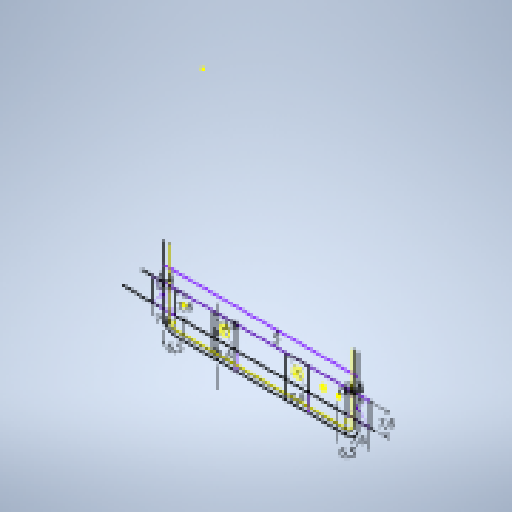
# Autodesk Inventor part: podstawa_rpi_board_2
Saved by Autodesk Inventor 2023.4 (Build 274418000, 418)
## iProperties
Created: 2024-09-15
Part Number: podstawa_rpi_board_2
Material: Generic
Document SubType Name: Modeling
Designer: komputer
Density: 1 g/cm^3
Appearance: Default
Author: komputer
Autodesk Inventor part; units mm, degrees
ref_plane "YZ Plane" through (0, 0, 0) normal (1, 0, 0) x (0, 1, 0)
ref_plane "XZ Plane" through (0, 0, 0) normal (0, 1, 0) x (-1, 0, 0)
ref_plane "XY Plane" through (0, 0, 0) normal (0, 0, 1) x (1, 0, 0)
sketch "Sketch1" plane through (0, 0, 0) normal (0, 0, 1) x (1, 0, 0)
  circle A0 centre (6.9875, -70.9975) radius 1.6 projected
  circle A1 centre (30.9875, -70.9975) radius 1.6 projected
  line L0 (49.2375, -55.2975) -> (49.2375, -76.7975) projected
  line L1 (-11.2625, -76.7975) -> (-11.2625, -55.2975) projected
  line L2 (47.2375, -78.7975) -> (-9.2625, -78.7975) projected
  line L3 (56.6281, -74.7975) -> (-26.6376, -74.7975)
  line L4 (54.4967, -67.1975) -> (-20.1835, -67.1975)
  line L5 (3.1875, -67.1975) -> (10.7875, -67.1975)
  line L6 (10.7875, -67.1975) -> (10.7875, -74.7975)
  line L7 (10.7875, -74.7975) -> (3.1875, -74.7975)
  line L8 (3.1875, -74.7975) -> (3.1875, -67.1975)
  line L9 (3.1875, -67.1975) -> (10.7875, -74.7975) construction
  line L10 (10.7875, -67.1975) -> (3.1875, -74.7975) construction
  line L11 (27.1875, -67.1975) -> (34.7875, -67.1975)
  line L12 (34.7875, -67.1975) -> (34.7875, -74.7975)
  line L13 (34.7875, -74.7975) -> (27.1875, -74.7975)
  line L14 (27.1875, -74.7975) -> (27.1875, -67.1975)
  line L15 (27.1875, -67.1975) -> (34.7875, -74.7975) construction
  line L16 (34.7875, -67.1975) -> (27.1875, -74.7975) construction
  line L17 (-16.8125, -67.1975) -> (-9.2125, -67.1975)
  line L18 (-9.2125, -67.1975) -> (-9.2125, -74.7975)
  line L19 (-9.2125, -74.7975) -> (-16.8125, -74.7975)
  line L20 (-16.8125, -74.7975) -> (-16.8125, -67.1975)
  line L21 (-16.8125, -67.1975) -> (-9.2125, -74.7975) construction
  line L22 (-9.2125, -67.1975) -> (-16.8125, -74.7975) construction
  line L23 (47.1875, -67.1975) -> (54.7875, -67.1975)
  line L24 (54.7875, -67.1975) -> (54.7875, -74.7975)
  line L25 (54.7875, -74.7975) -> (47.1875, -74.7975)
  line L26 (47.1875, -74.7975) -> (47.1875, -67.1975)
  line L27 (47.1875, -67.1975) -> (54.7875, -74.7975) construction
  line L28 (54.7875, -67.1975) -> (47.1875, -74.7975) construction
  circle A2 centre (39.4875, -70.9475) radius 0.9 projected
  circle A3 centre (44.4875, -70.9475) radius 0.75 projected
  circle A4 centre (-6.5125, -70.3475) radius 0.65 projected
  line L29 (49.4375, -67.1975) -> (49.4375, -74.7975)
  line L30 (-11.4625, -67.1975) -> (-11.4625, -74.7975)
  line L31 (51.0375, -67.1975) -> (51.0375, -74.7975)
  line L32 (-13.0625, -67.1975) -> (-13.0625, -74.7975)
  arc A5 (-11.2625, -76.7975) -> (-9.2625, -78.7975) centre (-9.2625, -76.7975) ccw projected
  arc A6 (47.2375, -78.7975) -> (49.2375, -76.7975) centre (47.2375, -76.7975) ccw projected
  line L33 (49.4375, -55.2975) -> (49.4375, -76.7975)
  arc A7 (47.2375, -78.9975) -> (49.4375, -76.7975) centre (47.2375, -76.7975) ccw
  line L34 (47.2375, -78.9975) -> (-9.2625, -78.9975)
  arc A8 (-11.4625, -76.7975) -> (-9.2625, -78.9975) centre (-9.2625, -76.7975) ccw
  line L35 (-11.4625, -76.7975) -> (-11.4625, -55.2975)
  line L36 (51.0375, -55.2975) -> (51.0375, -76.7975)
  arc A9 (47.2375, -80.5975) -> (51.0375, -76.7975) centre (47.2375, -76.7975) ccw
  line L37 (47.2375, -80.5975) -> (-9.2625, -80.5975)
  arc A10 (-13.0625, -76.7975) -> (-9.2625, -80.5975) centre (-9.2625, -76.7975) ccw
  line L38 (-13.0625, -76.7975) -> (-13.0625, -55.2975)
  line L39 (27.1875, -74.7975) -> (34.7875, -74.7975)
  line L40 (34.7875, -74.7975) -> (34.7875, -80.5975)
  line L41 (34.7875, -80.5975) -> (27.1875, -80.5975)
  line L42 (27.1875, -80.5975) -> (27.1875, -74.7975)
  line L43 (3.1875, -74.7975) -> (10.7875, -74.7975)
  line L44 (10.7875, -74.7975) -> (10.7875, -80.5975)
  line L45 (10.7875, -80.5975) -> (3.1875, -80.5975)
  line L46 (3.1875, -80.5975) -> (3.1875, -74.7975)
  line L47 (-13.0625, -67.1975) -> (51.0375, -67.1975)
  line L48 (51.0375, -67.1975) -> (51.0375, -62.1975)
  line L49 (51.0375, -62.1975) -> (-13.0625, -62.1975)
  line L50 (-13.0625, -62.1975) -> (-13.0625, -67.1975)
  point P0 (0, 0)
  point P1 (-13.0125, -70.9975)
  point P2 (50.9875, -70.9975)
  point P3 (3.1875, -78.9975)
  point P4 (-11.4625, -62.1975)
  point P5 (49.4375, -62.1975)
  point P6 (34.7875, -78.9975)
  point P7 (27.1875, -78.9975)
  point P8 (10.7875, -78.9975)
  dimension "d0" = 4
  dimension "d1" = 3.8
  dimension "d2" = 7.6
  dimension "d3" = 7.6
  dimension "d4" = 7.6
  dimension "d5" = 7.6
  dimension "d6" = 7.6
  dimension "d7" = 7.6
  dimension "d8" = 6.5
  dimension "d10" = 6.5
  dimension "d11" = 0.2
  dimension "d12" = 0.2
  dimension "d13" = 1.6
  dimension "d14" = 1.6
  dimension "d15" = 0.2
  dimension "d16" = 1.6
  dimension "d17" = 5
  constraints: 96 end point, 15 parallel, 13 point on line, 11 perpendicular, 8 horizontal, 8 midpoint, 8 point on circle, 4 centre point, 8 other
  measures "d0" distance between parallel lines of L2 L3
  measures "d1" distance from line of L4 A0.centre
  measures "d2" distance of L6.end L7.end
  measures "d3" distance of L12.end L13.end
  measures "d4" distance of L18.end L19.end
  measures "d5" distance of L17.end L18.end
  measures "d6" distance of L24.end L25.end
  measures "d7" distance of L23.end L24.end
  measures "d8" horizontal distance of point (50.988, -70.998) A3.centre
  measures "d10" horizontal distance of A4.centre point (-13.013, -70.998)
  measures "d11" distance between parallel lines of L30 L1
  measures "d12" distance between parallel lines of L0 L29
  measures "d13" distance between parallel lines of L31 L29
  measures "d14" distance between parallel lines of L30 L32
  measures "d15" distance between parallel lines of L0 L33
  measures "d16" distance between parallel lines of L33 L36
  measures "d17" distance between parallel lines of L49 L47
extrude "Extrusion1" add sketch "Sketch1" against normal blind 1.5 contours L4 L29 L3 L0 | L0 L3 L26 L4 | L49 L36 L4 L33 | L4 L31 L3 L29 | L4 L18 L3 L1 | L1 L3 L30 L4 | L35 L4 L38 L49 | L3 L36 A9 L37 L40 L34 A7 L33 | L12 L3 L14 L4 | L30 L3 L32 L4 | L40 L2 L42 L3 | L35 A8 L34 L46 L37 A10 L38 L3 | L4 L6 L3 L8 | L40 L34 L42 L2 | L3 L44 L2 L46 | L40 L37 L42 L34 | L2 L44 L34 L46 | L42 L37 L44 L34 | L34 L44 L37 L46
sketch "Sketch2" plane through (0, 0, 0) normal (0, 0, 1) x (1, 0, 0)
  line L0 (3.1875, -67.1975) -> (3.1875, -78.9975) projected
  line L1 (3.1875, -78.9975) -> (-9.2625, -78.9975) projected
  arc A0 (-11.4625, -76.7975) -> (-9.2625, -78.9975) centre (-9.2625, -76.7975) ccw projected
  line L2 (-11.4625, -76.7975) -> (-11.4625, -74.7975) projected
  line L3 (-11.4625, -74.7975) -> (-9.2125, -74.7975) projected
  line L4 (-9.2125, -74.7975) -> (-9.2125, -67.1975) projected
  line L5 (-9.2125, -67.1975) -> (-11.4625, -67.1975) projected
  line L6 (-11.4625, -67.1975) -> (-11.4625, -62.1975) projected
  line L7 (-11.4625, -62.1975) -> (-13.0625, -62.1975) projected
  line L8 (-13.0625, -62.1975) -> (-13.0625, -76.7975) projected
  arc A1 (-13.0625, -76.7975) -> (-9.2625, -80.5975) centre (-9.2625, -76.7975) ccw projected
  line L9 (-9.2625, -80.5975) -> (47.2375, -80.5975) projected
  arc A2 (47.2375, -80.5975) -> (51.0375, -76.7975) centre (47.2375, -76.7975) ccw projected
  line L10 (51.0375, -76.7975) -> (51.0375, -62.1975) projected
  line L11 (51.0375, -62.1975) -> (49.4375, -62.1975) projected
  line L12 (49.4375, -62.1975) -> (49.4375, -67.1975) projected
  line L13 (49.4375, -67.1975) -> (47.1875, -67.1975) projected
  line L14 (47.1875, -67.1975) -> (47.1875, -74.7975) projected
  line L15 (47.1875, -74.7975) -> (49.4375, -74.7975) projected
  line L16 (49.4375, -74.7975) -> (49.4375, -76.7975) projected
  arc A3 (47.2375, -78.9975) -> (49.4375, -76.7975) centre (47.2375, -76.7975) ccw projected
  line L17 (47.2375, -78.9975) -> (34.7875, -78.9975) projected
  line L18 (34.7875, -78.9975) -> (34.7875, -67.1975) projected
  line L19 (34.7875, -67.1975) -> (27.1875, -67.1975) projected
  line L20 (27.1875, -67.1975) -> (27.1875, -78.9975) projected
  line L21 (27.1875, -78.9975) -> (10.7875, -78.9975) projected
  line L22 (10.7875, -78.9975) -> (10.7875, -67.1975) projected
  line L23 (10.7875, -67.1975) -> (3.1875, -67.1975) projected
  circle A4 centre (30.9875, -70.9975) radius 1.6 projected
  circle A5 centre (6.9875, -70.9975) radius 1.6 projected
  line L24 (-11.4625, -76.7975) -> (-11.4625, -74.7975) projected
  line L25 (-11.4625, -67.1975) -> (-11.4625, -74.7975)
  line L26 (49.4375, -76.7975) -> (49.4375, -74.7975) projected
  line L27 (49.4375, -67.1975) -> (49.4375, -74.7975)
  line L28 (34.7875, -78.9975) -> (3.1875, -78.9975)
  line L29 (-9.2625, -80.5975) -> (47.2375, -80.5975) projected
  point P0 (0, 0)
  constraints: 6 end point, 2 vertical, 1 parallel
extrude "Extrusion2" add sketch "Sketch2" along normal blind 1.6 contours L28 L21 L17 A3 L16 L27 L12 L11 L10 A2 L9 A1 L8 L7 L6 L25 L2 A0 L1
sketch "Sketch3" plane through (0, 0, -1.5) normal (0, 0, -1) x (-1, 0, 0)
  line L0 (13.0625, -76.7975) -> (13.0625, -62.1975) projected
  arc A0 (9.2625, -80.5975) -> (13.0625, -76.7975) centre (9.2625, -76.7975) ccw projected
  line L1 (-47.2375, -80.5975) -> (9.2625, -80.5975) projected
  arc A1 (-51.0375, -76.7975) -> (-47.2375, -80.5975) centre (-47.2375, -76.7975) ccw projected
  line L2 (-51.0375, -62.1975) -> (-51.0375, -76.7975) projected
  line L3 (-49.4375, -62.1975) -> (-51.0375, -62.1975) projected
  line L4 (13.0625, -62.1975) -> (-51.0375, -62.1975)
  circle A2 centre (-6.9875, -70.9975) radius 1.6 projected
  circle A3 centre (-30.9875, -70.9975) radius 1.6 projected
  point P0 (0, 0)
  constraints: 2 end point, 1 horizontal
extrude "Extrusion3" add sketch "Sketch3" along normal blind 2
sketch "Sketch4" plane through (0, 0, -3.5) normal (0, 0, -1) x (-1, 0, 0)
  line L0 (13.0625, -62.1975) -> (-51.0375, -62.1975) projected
  line L1 (-51.0375, -62.1975) -> (-51.0375, -76.7975) projected
  arc A0 (-51.0375, -76.7975) -> (-47.2375, -80.5975) centre (-47.2375, -76.7975) ccw projected
  line L2 (-47.2375, -80.5975) -> (9.2625, -80.5975) projected
  arc A1 (9.2625, -80.5975) -> (13.0625, -76.7975) centre (9.2625, -76.7975) ccw projected
  line L3 (13.0625, -76.7975) -> (13.0625, -62.1975) projected
  circle A2 centre (-30.9875, -70.9975) radius 1.6 projected
  circle A3 centre (-6.9875, -70.9975) radius 1.6 projected
  point P0 (0, 0)
extrude "Extrusion4" add sketch "Sketch4" along normal blind 13.29 contours L3 A1 L2 A0 L1 L0 | A2 | A3
body "Solid1"
